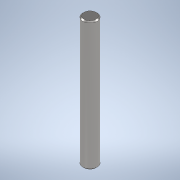
# Autodesk Inventor part: shaft
Saved by Autodesk Inventor 2020.1 (Build 241239000, 239)
## iProperties
Created: 2019-10-28
Part Number: shaft
Material: Stainless Steel
Document SubType Name: Modeling
Designer: agmle
Mass: 1.79698 g
Surface Area: 2.96455 cm^2
Volume: 0.224622 cm^3
Density: 8 g/cm^3
Appearance: Semi-Polished
Author: agmle
Autodesk Inventor part; units mm, degrees
ref_plane "YZ Plane" through (0, 0, 0) normal (1, 0, 0) x (0, 1, 0)
ref_plane "XZ Plane" through (0, 0, 0) normal (0, 1, 0) x (-1, 0, 0)
ref_plane "XY Plane" through (0, 0, 0) normal (0, 0, 1) x (1, 0, 0)
sketch "Sketch1" plane through (0, 0, 0) normal (0, 1, 0) x (-1, 0, 0)
  circle A0 centre (0, 0) radius 1.5875
  dimension "d0" = 3.175
  constraints: 1 centre point, 1 coincident
  measures "d0" diameter of A0
extrude "Extrusion1" add sketch "Sketch1" along normal blind 28.448
chamfer "Chamfer1" distance 0.254 angle 45 2 edges at (1.5875, 0, 0) (1.5875, 28.448, 0)
body "Solid1"
